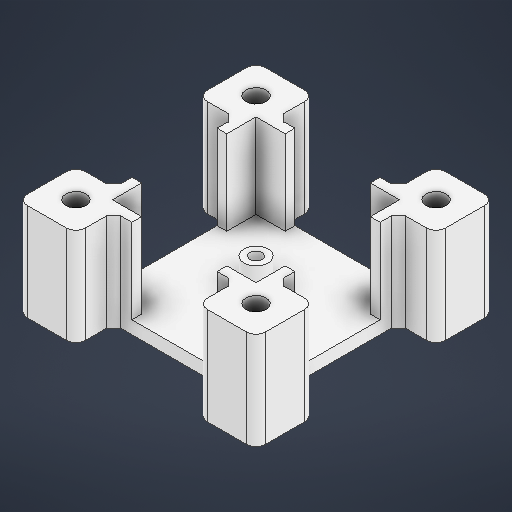
# Autodesk Inventor part: Electronica
Saved by Autodesk Inventor 2026.1 (Build 301233000, 233)
## iProperties
Created: 2025-11-15
Part Number: Electronica
Material: PLA
Document SubType Name: Modeling
Designer: vickh
Density: 1.3 g/cm^3
Appearance: Genérico
Mass: 145.55 g
Surface Area: 360.672 cm^2
Volume: 111.962 cm^3
Author: vickh
## iProperties of the stored document Electronica_3DPrint.ipt
Created: 2025-11-17
Part Number: Electronica_3DPrint
Material: Genérico
Document SubType Name: Modeling
Designer: usuario
Density: 1 g/cm^3
Appearance: Valor por defecto
Author: usuario
Autodesk Inventor part; units mm, degrees
ref_plane "YZ Plane" through (0, 0, 0) normal (1, 0, 0) x (0, 1, 0)
ref_plane "XZ Plane" through (0, 0, 0) normal (0, 1, 0) x (-1, 0, 0)
ref_plane "XY Plane" through (0, 0, 0) normal (0, 0, 1) x (1, 0, 0)
sketch "Boceto1" plane through (0, 0, 0) normal (0, 1, 0) x (-1, 0, 0)
  circle A0 centre (37, 37) radius 4.15
  line L0 (25, -33.5) -> (25, -49)
  line L1 (25, -49) -> (49, -49)
  line L2 (49, -49) -> (49, -25)
  line L3 (49, -25) -> (33.5, -25)
  line L4 (33.5, -25) -> (33.5, 25)
  line L5 (33.5, 25) -> (49, 25)
  line L6 (49, 25) -> (49, 49)
  line L7 (49, 49) -> (25, 49)
  line L8 (25, 49) -> (25, 33.5)
  line L9 (25, 33.5) -> (-25, 33.5)
  line L10 (-25, 33.5) -> (-25, 49)
  line L11 (-25, 49) -> (-49, 49)
  line L12 (-49, 49) -> (-49, 25)
  line L13 (-49, 25) -> (-33.5, 25)
  line L14 (-33.5, 25) -> (-33.5, -25)
  line L15 (-33.5, -25) -> (-49, -25)
  line L16 (-49, -25) -> (-49, -49)
  line L17 (-49, -49) -> (-25, -49)
  line L18 (-25, -49) -> (-25, -33.5)
  line L19 (-25, -33.5) -> (25, -33.5)
  circle A1 centre (0, 0) radius 5
  line L20 (49, -49) -> (-49, -49) construction
  line L21 (-49, -49) -> (-49, 49)
  line L22 (-49, 49) -> (49, 49) construction
  line L23 (49, 49) -> (49, -49) construction
  line L24 (49, -49) -> (25.0011, -49) construction
  line L25 (25.0011, -49) -> (25.0011, -25) construction
  line L26 (49, -25) -> (49, -49) construction
  line L27 (0, -49) -> (0, 49) construction
  line L28 (49, 0) -> (-49, 0) construction
  line L29 (49, 49) -> (25, 49) construction
  line L30 (25, 49) -> (25, 25) construction
  line L31 (25, 25) -> (49, 25) construction
  line L32 (49, 25) -> (49, 49) construction
  line L33 (49, 49) -> (25, 25) construction
  line L34 (49, 25) -> (25, 49) construction
  circle A2 centre (-37, 37) radius 4.15
  circle A3 centre (-37, -37) radius 4.15
  circle A4 centre (37, -37) radius 4.15
  line L35 (29.5, 29.5) -> (-29.5, 29.5)
  line L36 (-29.5, 29.5) -> (-29.5, -29.5)
  line L37 (-29.5, -29.5) -> (29.5, -29.5)
  line L38 (29.5, -29.5) -> (29.5, 29.5)
  line L39 (29.5, 29.5) -> (-29.5, -29.5) construction
  line L40 (-29.5, 29.5) -> (29.5, -29.5) construction
  circle A5 centre (0, 0) radius 2.5
  point P0 (33.5, 0)
  point P1 (0, -33.5)
  point P2 (0, 33.5)
  point P3 (-33.5, 0)
  dimension "d0" = 33.5
  dimension "d1" = 33.5
  dimension "d4" = 8.3
  dimension "d6" = 49
  dimension "d7" = 49
  dimension "d8" = 98
  dimension "d9" = 98
  dimension "d10" = 15.5
  dimension "d11" = 15.5
  dimension "d12" = 15.5
  dimension "d13" = 15.5
  dimension "d14" = 50
  dimension "d15" = 50
  dimension "d16" = 15.5
  dimension "d17" = 15.5
  dimension "d18" = 15.5
  dimension "d19" = 50
  dimension "d20" = 25
  dimension "d21" = 25
  dimension "d22" = 25
  dimension "d23" = 25
  dimension "d24" = 10
  dimension "d26" = 8.5
  dimension "d27" = 8.5
  dimension "d28" = 24
  dimension "d29" = 15.5
  dimension "d30" = 24
  dimension "d31" = 8.5
  dimension "d32" = 24
  dimension "d33" = 24
  dimension "d36" = 360
  dimension "d41" = 4
  dimension "d46" = 5
  dimension "d49" = 4
  constraints: 82 end point, 11 midpoint, 7 horizontal, 7 parallel, 7 vertical, 6 centre point, 4 perpendicular, 3 coincident, 3 point on line, 9 other
  measures "d0" distance of point (0, 0) point (33.5, 0)
  measures "d1" distance from line of point (0, 0) L14
  measures "d4" diameter of A0
  measures "d6" distance of point (0, 0) L28.end
  measures "d7" distance from line of L20 point (0, 0)
  measures "d8" distance of L2.start L20.end
  measures "d9" distance of L20.end L12.start
  measures "d10" distance between parallel lines of L22 L9
  measures "d11" distance between parallel lines of L23 L4
  measures "d12" distance between parallel lines of L20 L19
  measures "d13" distance of L14.end L15.end
  measures "d14" distance of L19.start L19.end
  measures "d15" distance of L9.start L9.end
  measures "d16" distance of L7.end L9.start
  measures "d17" distance of L9.end L11.start
  measures "d18" distance of L13.start L14.start
  measures "d19" distance of L14.start L14.end
  measures "d20" distance from line of point (0, 0) L15
  measures "d21" distance from line of L3 point (0, 0)
  measures "d22" distance from line of point (0, 0) L5
  measures "d23" distance from line of point (0, 0) L13
  measures "d24" diameter of A1
  measures "d26" horizontal distance of L14.end L19.start
  measures "d27" distance from line of L10 L14.start
  measures "d28" distance of L5.end L6.end
  measures "d29" distance of L18.start L19.start
  measures "d30" distance of L6.end L7.end
  measures "d31" horizontal distance of L4.start L19.end
  measures "d32" distance of L31.end L30.end
  measures "d33" distance of L30.end L29.end
  measures "d41" distance between parallel lines of L37 L19
  measures "d46" diameter of A5
  measures "d49" distance between parallel lines of L4 L38
extrude "Extrusión1" add sketch "Boceto1" along normal blind 40 contours L19 L18 L17 L16 L15 L14 L13 L12 L11 L10 L9 L8 L7 L6 L5 L4 L3 L2 L1 L0
extrude "Extrusión2" add sketch "Boceto1" along normal blind 5.3 contours L38 L37 L36 L35
extrude "Extrusión3" add sketch "Boceto1" along normal blind 20 contours A1
extrude "Extrusión4" add sketch "Boceto1" along normal blind 10 contours A5
sketch "Boceto2" plane through (0, 40, 0) normal (0, 1, 0) x (1, 0, 0)
  line L0 (33.5, -25) -> (33.5, 25) projected
  line L1 (-33.5, 17.5) -> (33.5, 17.5)
  line L2 (33.5, 17.5) -> (33.5, -17.5)
  line L3 (33.5, -17.5) -> (-33.5, -17.5)
  line L4 (-33.5, -17.5) -> (-33.5, 17.5)
  circle A0 centre (0, 0) radius 2.5 projected
  line L5 (-33.5, 17.5) -> (33.5, -17.5) construction
  line L6 (33.5, 17.5) -> (-33.5, -17.5) construction
  line L7 (17.5, 33.5) -> (-17.5, 33.5)
  line L8 (-17.5, 33.5) -> (-17.5, -33.5)
  line L9 (-17.5, -33.5) -> (17.5, -33.5)
  line L10 (17.5, -33.5) -> (17.5, 33.5)
  line L11 (17.5, 33.5) -> (-17.5, -33.5) construction
  line L12 (-17.5, 33.5) -> (17.5, -33.5) construction
  line L13 (-25, -33.5) -> (25, -33.5) projected
  line L14 (29.5, 29.5) -> (29.5, -29.5) projected
  line L15 (-29.5, 29.5) -> (29.5, 29.5) projected
  line L16 (-29.5, -29.5) -> (-29.5, 29.5) projected
  line L17 (29.5, -29.5) -> (-29.5, -29.5) projected
  circle A1 centre (0, 0) radius 5 projected
  point P0 (-17.5, 29.5)
  point P1 (17.5, 29.5)
  point P2 (-29.5, -17.5)
  point P3 (-29.5, 17.5)
  point P4 (17.5, -29.5)
  point P5 (-17.5, -29.5)
  point P6 (29.5, 17.5)
  point P7 (29.5, -17.5)
  dimension "d50" = 35
  dimension "d51" = 35
  constraints: 24 end point, 4 midpoint, 4 parallel, 2 horizontal, 2 perpendicular, 1 collinear, 1 point on line
  measures "d50" distance of L1.end L2.end
  measures "d51" distance of L8.end L9.end
extrude "Extrusión5" cut sketch "Boceto2" against normal up to surface (34.7 mm away) contours L3 L14 L1 L0 | L10 L9 L8 L17 | L15 L8 L7 L10 | L3 L4 L1 L16
fillet "Empalme1" radius 4 12 edges at (49, 20, 49) (49, 20, -49) (49, 20, 25) (25, 20, -49) (-25, 20, -49) (-49, 20, -49) (-49, 20, -25) (-49, 20, 25) (-49, 20, 49) (-25, 20, 49) (25, 20, 49) (49, 20, -25)
chamfer "Chaflán1" distance 3 angle 45 8 edges at (33.5, 20, 25) (33.5, 20, -25) (25, 20, -33.5) (-25, 20, -33.5) (-33.5, 20, -25) (-33.5, 20, 25) (-25, 20, 33.5) (25, 20, 33.5)
